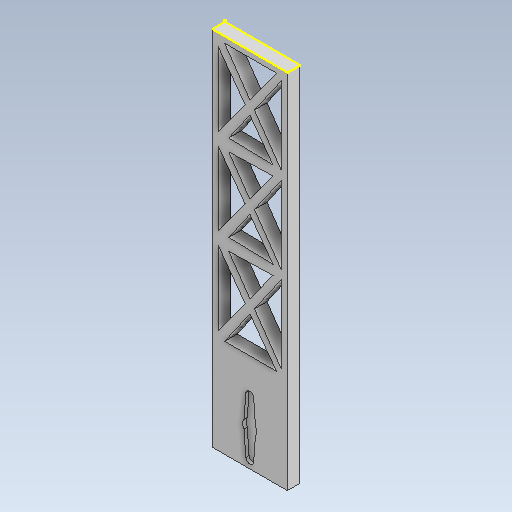
# Autodesk Inventor part: First Leg
Saved by Autodesk Inventor 2020.2 (Build 242310000, 310)
## iProperties
Created: 2020-03-02
Part Number: First Leg
Material: Generic
Document SubType Name: Modeling
Designer: othscs164
Density: 1 g/cm^3
Appearance: Default
Author: othscs164
Autodesk Inventor part; units mm, degrees
ref_plane "YZ Plane" through (0, 0, 0) normal (1, 0, 0) x (0, 1, 0)
ref_plane "XZ Plane" through (0, 0, 0) normal (0, 1, 0) x (-1, 0, 0)
ref_plane "XY Plane" through (0, 0, 0) normal (0, 0, 1) x (1, 0, 0)
sketch "Sketch1" plane through (0, 0, 0) normal (0, 0, 1) x (1, 0, 0)
  line L0 (0, 0) -> (38.1, 0)
  line L1 (38.1, 0) -> (38.1, 203.2)
  line L2 (38.1, 203.2) -> (0, 203.2)
  line L3 (0, 203.2) -> (0, 0)
  dimension "d0" = 38.1
  dimension "d1" = 203.2
  constraints: 8 end point, 2 parallel, 1 horizontal, 1 perpendicular
  measures "d0" distance of L2.end L1.end
  measures "d1" distance of L1.end L0.end
extrude "Extrusion1" add sketch "Sketch1" along normal blind 6.35
sketch "Sketch2" plane through (0, 0, 6.35) normal (0, 0, 1) x (1, 0, 0)
  line L0 (21.925, 35.9667) -> (21.0447, 23.9538)
  line L1 (17.0553, 23.9538) -> (16.175, 35.9667)
  line L2 (21.925, 40.2333) -> (21.0447, 52.2462)
  line L3 (17.0553, 52.2462) -> (16.175, 40.2333)
  arc A0 (21.925, 35.9667) -> (21.925, 40.2333) centre (19.05, 38.1) ccw
  arc A1 (16.175, 40.2333) -> (16.175, 35.9667) centre (19.05, 38.1) ccw
  arc A2 (17.0553, 23.9538) -> (21.0447, 23.9538) centre (19.05, 24.1) ccw
  arc A3 (21.0447, 52.2462) -> (17.0553, 52.2462) centre (19.05, 52.1) ccw
  line L4 (0, 0) -> (38.1, 0) projected
  line L5 (38.1, 0) -> (38.1, 38.1)
  line L6 (38.1, 0) -> (38.1, 203.2) projected
  line L7 (38.1, 0) -> (76.2, 0) construction
  line L8 (38.1, 38.1) -> (19.05, 38.1)
  line L9 (20.546, 52.2096) -> (21.4374, 40.046)
  arc A4 (21.4374, 36.154) -> (21.4374, 40.046) centre (19.05, 38.1) ccw
  line L10 (21.4374, 36.154) -> (20.546, 23.9904)
  arc A5 (17.554, 23.9904) -> (20.546, 23.9904) centre (19.05, 24.1) ccw
  line L11 (17.554, 23.9904) -> (16.6626, 36.154)
  arc A6 (16.6626, 40.046) -> (16.6626, 36.154) centre (19.05, 38.1) ccw
  line L12 (16.6626, 40.046) -> (17.554, 52.2096)
  arc A7 (20.546, 52.2096) -> (17.554, 52.2096) centre (19.05, 52.1) ccw
  dimension "d4" = 38.1
  dimension "d5" = 90
  dimension "d6" = 19.05
  dimension "d7" = 270
  dimension "d8" = 0.5
  constraints: 22 end point, 16 point on circle, 8 centre point, 2 parallel, 2 perpendicular, 1 collinear, 1 horizontal, 7 other
  measures "d4" distance of L4.end L5.end
  measures "d5" angle of L7 L5
  measures "d6" distance of L5.end L8.end
  measures "d8" distance between parallel lines of L2 L9
extrude "Extrusion2" cut sketch "Sketch2" against normal blind 1.651 contours L9 A4 L10 A5 L11 A6 L12 A7
sketch "Sketch3" plane through (0, 0, 6.35) normal (0, 0, 1) x (1, 0, 0)
  line L0 (21.4374, 36.154) -> (20.546, 23.9904) projected
  arc A0 (17.554, 23.9904) -> (20.546, 23.9904) centre (19.05, 24.1) ccw projected
  line L1 (17.554, 23.9904) -> (16.6626, 36.154) projected
  arc A1 (16.6626, 40.046) -> (16.6626, 36.154) centre (19.05, 38.1) ccw projected
  line L2 (16.6626, 40.046) -> (17.554, 52.2096) projected
  arc A2 (20.546, 52.2096) -> (17.554, 52.2096) centre (19.05, 52.1) ccw projected
  line L3 (20.546, 52.2096) -> (21.4374, 40.046) projected
  arc A3 (21.4374, 36.154) -> (21.4374, 40.046) centre (19.05, 38.1) ccw projected
  line L4 (0, 0) -> (38.1, 0) projected
  line L5 (38.1, 0) -> (38.1, 203.2) projected
  line L6 (38.1, 203.2) -> (0, 203.2) projected
  line L7 (0, 203.2) -> (0, 0) projected
  line L8 (0, 203.2) -> (0, 0) projected
  line L9 (0, 66.3224) -> (38.1, 66.3224)
  line L10 (38.1, 0) -> (38.1, 203.2) projected
  line L11 (0, 66.3224) -> (0, 203.2)
  line L12 (38.1, 203.2) -> (0, 203.2) projected
  line L13 (0, 203.2) -> (38.1, 203.2)
  line L14 (38.1, 203.2) -> (38.1, 66.3224)
  line L15 (3.175, 200.025) -> (3.175, 69.4974)
  line L16 (3.175, 69.4974) -> (34.925, 69.4974)
  line L17 (34.925, 69.4974) -> (34.925, 200.025)
  line L18 (34.925, 200.025) -> (3.175, 200.025)
  line L19 (34.925, 69.4974) -> (34.925, 113.0076)
  line L20 (34.925, 113.0076) -> (3.175, 113.0076)
  line L21 (34.925, 69.4974) -> (3.175, 113.0076)
  line L22 (34.925, 113.0076) -> (3.175, 69.4974)
  line L23 (3.175, 69.4974) -> (19.05, 91.2525)
  line L24 (3.175, 113.0076) -> (19.05, 91.2525)
  line L25 (3.175, 69.4974) -> (3.175, 113.0076)
  line L26 (3.175, 113.0076) -> (34.925, 113.0076)
  line L27 (19.05, 91.2525) -> (34.925, 113.0076)
  line L28 (34.925, 69.4974) -> (19.05, 91.2525)
  line L29 (34.925, 69.4974) -> (34.925, 113.0076)
  line L30 (34.925, 69.4974) -> (3.175, 69.4974)
  line L31 (3.175, 69.4974) -> (3.175, 113.0076)
  line L32 (3.175, 113.0076) -> (34.925, 113.0076)
  line L33 (3.175, 69.4974) -> (3.175, 72.6724)
  line L34 (3.175, 72.6724) -> (32.6082, 113.0076)
  line L35 (21.925, 35.9667) -> (21.0447, 23.9538)
  line L36 (17.0553, 23.9538) -> (16.175, 35.9667)
  line L37 (21.925, 40.2333) -> (21.0447, 52.2462)
  line L38 (17.0553, 52.2462) -> (16.175, 40.2333)
  arc A4 (21.925, 35.9667) -> (21.925, 40.2333) centre (19.05, 38.1) ccw
  arc A5 (16.175, 40.2333) -> (16.175, 35.9667) centre (19.05, 38.1) ccw
  arc A6 (17.0553, 23.9538) -> (21.0447, 23.9538) centre (19.05, 24.1) ccw
  arc A7 (21.0447, 52.2462) -> (17.0553, 52.2462) centre (19.05, 52.1) ccw
  line L39 (34.925, 113.0076) -> (34.925, 110.6962)
  line L40 (3.175, 69.4974) -> (6.35, 69.4974)
  line L41 (6.35, 69.4974) -> (34.925, 110.6962)
  line L42 (3.175, 113.0076) -> (3.175, 109.8326)
  line L43 (3.175, 113.0076) -> (6.35, 113.0076) construction
  line L44 (34.925, 69.4974) -> (32.6136, 69.4974)
  line L45 (34.925, 69.4974) -> (37.2364, 69.4974) construction
  line L46 (32.6136, 69.4974) -> (3.175, 109.8326)
  line L47 (34.925, 69.4974) -> (34.925, 71.8088)
  line L48 (3.175, 113.0076) -> (6.35, 113.0076)
  line L49 (6.35, 113.0076) -> (34.925, 71.8088)
  line L50 (3.175, 69.4974) -> (3.175, 113.0076)
  line L51 (34.925, 69.4974) -> (34.925, 113.0076)
  line L52 (34.925, 156.5178) -> (3.175, 156.5178)
  line L53 (34.925, 113.0076) -> (34.925, 156.5178)
  line L54 (34.925, 113.0076) -> (32.6136, 113.0076)
  line L55 (34.925, 113.0076) -> (34.925, 115.319)
  line L56 (34.925, 113.0076) -> (34.925, 156.5178)
  line L57 (34.925, 156.5178) -> (34.925, 154.2064)
  line L58 (34.925, 113.0076) -> (34.925, 156.5178)
  line L59 (19.05, 134.7627) -> (34.925, 156.5178)
  line L60 (3.175, 156.5178) -> (34.925, 156.5178)
  line L61 (3.175, 156.5178) -> (34.925, 156.5178)
  line L62 (3.175, 156.5178) -> (19.05, 134.7627)
  line L63 (3.175, 156.5178) -> (6.35, 156.5178)
  line L64 (3.175, 156.5178) -> (6.35, 156.5178) construction
  line L65 (3.175, 156.5178) -> (3.175, 153.3428)
  line L66 (3.175, 116.1826) -> (32.6082, 156.5178)
  line L67 (6.35, 156.5178) -> (34.925, 115.319)
  line L68 (34.925, 113.0076) -> (3.175, 156.5178)
  line L69 (34.925, 156.5178) -> (3.175, 113.0076)
  line L70 (3.175, 113.0076) -> (3.175, 156.5178)
  line L71 (3.175, 113.0076) -> (3.175, 156.5178)
  line L72 (3.175, 113.0076) -> (3.175, 156.5178)
  line L73 (6.35, 113.0076) -> (34.925, 154.2064)
  line L74 (32.6136, 113.0076) -> (3.175, 153.3428)
  line L75 (3.175, 113.0076) -> (34.925, 113.0076)
  line L76 (34.925, 113.0076) -> (19.05, 134.7627)
  line L77 (34.925, 113.0076) -> (3.175, 113.0076)
  line L78 (3.175, 113.0076) -> (19.05, 134.7627)
  line L79 (3.175, 113.0076) -> (3.175, 116.1826)
  line L80 (3.175, 113.0076) -> (6.35, 113.0076)
  line L81 (34.925, 200.028) -> (3.175, 200.028)
  line L82 (34.925, 156.5178) -> (34.925, 200.028)
  line L83 (34.925, 156.5178) -> (32.6136, 156.5178)
  line L84 (34.925, 156.5178) -> (34.925, 158.8292)
  line L85 (34.925, 156.5178) -> (34.925, 200.028)
  line L86 (34.925, 200.028) -> (34.925, 197.7166)
  line L87 (34.925, 156.5178) -> (34.925, 200.028)
  line L88 (19.05, 178.2729) -> (34.925, 200.028)
  line L89 (3.175, 200.028) -> (34.925, 200.028)
  line L90 (3.175, 200.028) -> (34.925, 200.028)
  line L91 (3.175, 200.028) -> (19.05, 178.2729)
  line L92 (3.175, 200.028) -> (6.35, 200.028)
  line L93 (3.175, 200.028) -> (6.35, 200.028) construction
  line L94 (3.175, 200.028) -> (3.175, 196.853)
  line L95 (3.175, 159.6928) -> (32.6082, 200.028)
  line L96 (6.35, 200.028) -> (34.925, 158.8292)
  line L97 (34.925, 156.5178) -> (3.175, 200.028)
  line L98 (34.925, 200.028) -> (3.175, 156.5178)
  line L99 (3.175, 156.5178) -> (3.175, 200.028)
  line L100 (3.175, 156.5178) -> (3.175, 200.028)
  line L101 (3.175, 156.5178) -> (3.175, 200.028)
  line L102 (6.35, 156.5178) -> (34.925, 197.7166)
  line L103 (32.6136, 156.5178) -> (3.175, 196.853)
  line L104 (3.175, 156.5178) -> (34.925, 156.5178)
  line L105 (34.925, 156.5178) -> (19.05, 178.2729)
  line L106 (34.925, 156.5178) -> (3.175, 156.5178)
  line L107 (3.175, 156.5178) -> (19.05, 178.2729)
  line L108 (3.175, 156.5178) -> (3.175, 159.6928)
  line L109 (3.175, 156.5178) -> (6.35, 156.5178)
  line L110 (34.925, 115.319) -> (3.175, 116.1826)
  line L111 (3.175, 109.8326) -> (34.925, 110.6962)
  line L112 (34.925, 158.8292) -> (3.175, 159.6928)
  line L113 (3.175, 153.3428) -> (34.925, 154.2064)
  dimension "d12" = 3.175
  dimension "d13" = 43.5102
  dimension "d14" = 3.175
  dimension "d17" = 2.3114
  dimension "d18" = 3.175
  dimension "d19" = 3.175
  dimension "d20" = 270
  dimension "d21" = 2.3114
  dimension "d22" = 180
  dimension "d23" = 2.3114
  dimension "d24" = 3.175
  dimension "d27" = 43.5102
  constraints: 206 end point, 19 point on line, 10 perpendicular, 8 collinear, 8 point on circle, 4 centre point, 4 parallel, 3 horizontal, 2 equal length, 1 midpoint, 1 vertical, 87 other
  measures "d12" distance between parallel lines of L11 L15
  measures "d13" distance of L16.end L19.end
  measures "d14" distance of L15.end L33.end
  measures "d17" distance of L19.end L39.end
  measures "d18" distance of L15.end L40.end
  measures "d19" distance of L20.end L42.end
  measures "d21" distance of L16.end L44.end
  measures "d22" angle of L45 L44
  measures "d23" distance of L16.end L47.end
  measures "d24" distance of L20.end L43.end
  measures "d27" distance of L15.end L69.end
extrude "Extrusion3" cut sketch "Sketch3" against normal blind 1.651 contours L35 A6 L36 A5 L38 A7 L37 A4
sketch "Sketch4" plane through (0, 0, 6.35) normal (0, 0, 1) x (1, 0, 0)
  line L0 (0, 66.3224) -> (38.1, 66.3224)
  line L1 (0, 66.3224) -> (0, 203.2)
  line L2 (0, 203.2) -> (38.1, 203.2)
  line L3 (38.1, 203.2) -> (38.1, 66.3224)
  line L4 (3.175, 200.025) -> (3.175, 69.4974)
  line L5 (3.175, 69.4974) -> (34.925, 69.4974)
  line L6 (34.925, 69.4974) -> (34.925, 200.025)
  line L7 (34.925, 200.025) -> (3.175, 200.025)
  line L8 (34.925, 69.4974) -> (34.925, 113.0076)
  line L9 (34.925, 113.0076) -> (3.175, 113.0076)
  line L10 (34.925, 69.4974) -> (3.175, 113.0076)
  line L11 (34.925, 113.0076) -> (3.175, 69.4974)
  line L12 (3.175, 69.4974) -> (19.05, 91.2525)
  line L13 (3.175, 113.0076) -> (19.05, 91.2525)
  line L14 (3.175, 69.4974) -> (3.175, 113.0076)
  line L15 (3.175, 113.0076) -> (34.925, 113.0076)
  line L16 (19.05, 91.2525) -> (34.925, 113.0076)
  line L17 (34.925, 69.4974) -> (19.05, 91.2525)
  line L18 (34.925, 69.4974) -> (34.925, 113.0076)
  line L19 (34.925, 69.4974) -> (3.175, 69.4974)
  line L20 (3.175, 69.4974) -> (3.175, 113.0076)
  line L21 (3.175, 113.0076) -> (34.925, 113.0076)
  line L22 (3.175, 69.4974) -> (3.175, 72.6724)
  line L23 (3.175, 72.6724) -> (32.6082, 113.0076)
  line L24 (34.925, 113.0076) -> (34.925, 110.6962)
  line L25 (3.175, 69.4974) -> (6.35, 69.4974)
  line L26 (6.35, 69.4974) -> (34.925, 110.6962)
  line L27 (3.175, 113.0076) -> (3.175, 109.8326)
  line L28 (3.175, 113.0076) -> (6.35, 113.0076) construction
  line L29 (34.925, 69.4974) -> (32.6136, 69.4974)
  line L30 (34.925, 69.4974) -> (37.2364, 69.4974) construction
  line L31 (32.6136, 69.4974) -> (3.175, 109.8326)
  line L32 (34.925, 69.4974) -> (34.925, 71.8088)
  line L33 (3.175, 113.0076) -> (6.35, 113.0076)
  line L34 (6.35, 113.0076) -> (34.925, 71.8088)
  line L35 (3.175, 69.4974) -> (3.175, 113.0076)
  line L36 (34.925, 69.4974) -> (34.925, 113.0076)
  line L37 (34.925, 156.5178) -> (3.175, 156.5178)
  line L38 (34.925, 113.0076) -> (34.925, 156.5178)
  line L39 (34.925, 113.0076) -> (32.6136, 113.0076)
  line L40 (34.925, 113.0076) -> (34.925, 115.319)
  line L41 (34.925, 113.0076) -> (34.925, 156.5178)
  line L42 (34.925, 156.5178) -> (34.925, 154.2064)
  line L43 (34.925, 113.0076) -> (34.925, 156.5178)
  line L44 (19.05, 134.7627) -> (34.925, 156.5178)
  line L45 (3.175, 156.5178) -> (34.925, 156.5178)
  line L46 (3.175, 156.5178) -> (34.925, 156.5178)
  line L47 (3.175, 156.5178) -> (19.05, 134.7627)
  line L48 (3.175, 156.5178) -> (6.35, 156.5178)
  line L49 (3.175, 156.5178) -> (6.35, 156.5178) construction
  line L50 (3.175, 156.5178) -> (3.175, 153.3428)
  line L51 (3.175, 116.1826) -> (32.6082, 156.5178)
  line L52 (6.35, 156.5178) -> (34.925, 115.319)
  line L53 (34.925, 113.0076) -> (3.175, 156.5178)
  line L54 (34.925, 156.5178) -> (3.175, 113.0076)
  line L55 (3.175, 113.0076) -> (3.175, 156.5178)
  line L56 (3.175, 113.0076) -> (3.175, 156.5178)
  line L57 (3.175, 113.0076) -> (3.175, 156.5178)
  line L58 (6.35, 113.0076) -> (34.925, 154.2064)
  line L59 (32.6136, 113.0076) -> (3.175, 153.3428)
  line L60 (3.175, 113.0076) -> (34.925, 113.0076)
  line L61 (34.925, 113.0076) -> (19.05, 134.7627)
  line L62 (34.925, 113.0076) -> (3.175, 113.0076)
  line L63 (3.175, 113.0076) -> (19.05, 134.7627)
  line L64 (3.175, 113.0076) -> (3.175, 116.1826)
  line L65 (3.175, 113.0076) -> (6.35, 113.0076)
  line L66 (34.925, 200.028) -> (3.175, 200.028)
  line L67 (34.925, 156.5178) -> (34.925, 200.028)
  line L68 (34.925, 156.5178) -> (32.6136, 156.5178)
  line L69 (34.925, 156.5178) -> (34.925, 158.8292)
  line L70 (34.925, 156.5178) -> (34.925, 200.028)
  line L71 (34.925, 200.028) -> (34.925, 197.7166)
  line L72 (34.925, 156.5178) -> (34.925, 200.028)
  line L73 (19.05, 178.2729) -> (34.925, 200.028)
  line L74 (3.175, 200.028) -> (34.925, 200.028)
  line L75 (3.175, 200.028) -> (34.925, 200.028)
  line L76 (3.175, 200.028) -> (19.05, 178.2729)
  line L77 (3.175, 200.028) -> (6.35, 200.028)
  line L78 (3.175, 200.028) -> (6.35, 200.028) construction
  line L79 (3.175, 200.028) -> (3.175, 196.853)
  line L80 (3.175, 159.6928) -> (32.6082, 200.028)
  line L81 (6.35, 200.028) -> (34.925, 158.8292)
  line L82 (34.925, 156.5178) -> (3.175, 200.028)
  line L83 (34.925, 200.028) -> (3.175, 156.5178)
  line L84 (3.175, 156.5178) -> (3.175, 200.028)
  line L85 (3.175, 156.5178) -> (3.175, 200.028)
  line L86 (3.175, 156.5178) -> (3.175, 200.028)
  line L87 (6.35, 156.5178) -> (34.925, 197.7166)
  line L88 (32.6136, 156.5178) -> (3.175, 196.853)
  line L89 (3.175, 156.5178) -> (34.925, 156.5178)
  line L90 (34.925, 156.5178) -> (19.05, 178.2729)
  line L91 (34.925, 156.5178) -> (3.175, 156.5178)
  line L92 (3.175, 156.5178) -> (19.05, 178.2729)
  line L93 (3.175, 156.5178) -> (3.175, 159.6928)
  line L94 (3.175, 156.5178) -> (6.35, 156.5178)
  line L95 (34.925, 115.319) -> (3.175, 116.1826)
  line L96 (3.175, 109.8326) -> (34.925, 110.6962)
  line L97 (34.925, 158.8292) -> (3.175, 159.6928)
  line L98 (3.175, 153.3428) -> (34.925, 154.2064)
  point P0 (0, 0)
  point P1 (30.8404, 110.5851)
  point P2 (8.4526, 109.9761)
  point P3 (19.1458, 94.5588)
  point P4 (34.925, 110.6962)
  point P5 (21.4391, 91.2525)
  point P6 (19.1473, 87.9482)
  point P7 (16.7344, 91.2542)
  point P8 (3.175, 109.8326)
  point P9 (21.4391, 134.7627)
  point P10 (30.8456, 115.4299)
  point P11 (19.1473, 131.4584)
  point P12 (8.4526, 116.039)
  point P13 (16.7344, 134.7644)
  point P14 (19.1458, 138.069)
  point P15 (30.8404, 154.0953)
  point P16 (8.4526, 153.4863)
  point P17 (19.1473, 174.9686)
  point P18 (8.4526, 159.5492)
  point P19 (30.8456, 158.9401)
  point P20 (16.7344, 178.2746)
  point P21 (3.175, 196.853)
  point P22 (19.1458, 181.5792)
  point P23 (32.606, 200.025)
  point P24 (6.352, 200.025)
  point P25 (21.4391, 178.2729)
  dimension "d36" = 3.175
  dimension "d37" = 43.5102
  dimension "d38" = 3.175
  dimension "d39" = 2.3114
  dimension "d40" = 3.175
  dimension "d41" = 3.175
  dimension "d42" = 270
  dimension "d43" = 2.3114
  dimension "d44" = 180
  dimension "d45" = 2.3114
  dimension "d46" = 3.175
  dimension "d47" = 43.5102
  constraints: 198 end point, 17 point on line, 8 perpendicular, 7 collinear, 3 horizontal, 3 parallel, 2 equal length, 1 midpoint, 1 vertical, 87 other
  measures "d36" distance between parallel lines of L1 L4
  measures "d37" distance of L6.start L15.end
  measures "d38" distance of L4.end L23.start
  measures "d39" distance of L15.end L26.end
  measures "d40" distance of L4.end L26.start
  measures "d41" distance of L15.start L31.end
  measures "d43" distance of L6.start L31.start
  measures "d44" angle of L30 L29
  measures "d45" distance of L6.start L34.end
  measures "d46" distance of L15.start L34.start
  measures "d47" distance of L4.end L60.start
extrude "Extrusion4" cut sketch "Sketch4" against normal up to surface (6.35 mm away) contours L88 L80 L4 | L7 L80 L81 | L59 L51 L4 | L87 L88 L97 | L87 L6 L81 | L98 L51 L52 | L6 L52 L58 | L31 L23 L4 | L58 L59 L95 | L96 L23 L34 | L6 L34 L26 | L26 L31 L5
sketch "Sketch5" plane through (0, 0, 6.35) normal (0, 0, 1) x (1, 0, 0)
  line L0 (0, 0) -> (38.1, 0) projected
  line L1 (0, 0) -> (0, 20)
  line L2 (0, 203.2) -> (0, 0) projected
  line L3 (0, 0) -> (20, 0) construction
  line L4 (0, 20) -> (38.1, 20)
  line L5 (38.1, 0) -> (38.1, 203.2) projected
  line L6 (38.1, 0) -> (38.1, 20)
  line L7 (38.1, 0) -> (0, 0)
  dimension "d51" = 20
  dimension "d52" = 270
  constraints: 10 end point, 4 perpendicular, 1 collinear, 1 horizontal, 1 point on line
  measures "d51" distance of L0.start L1.end
extrude "Extrusion5" cut sketch "Sketch5" against normal up to surface (6.35 mm away)
sketch "Sketch6" plane through (0, 203.2, 0) normal (0, 1, 0) x (1, 0, 0)
  line L0 (38.1, 0) -> (0, 0) projected
  line L1 (0, 0) -> (0, -6.35) projected
  line L2 (38.1, -6.35) -> (0, -6.35) projected
  line L3 (38.1, 0) -> (38.1, -6.35) projected
body "Solid1"
